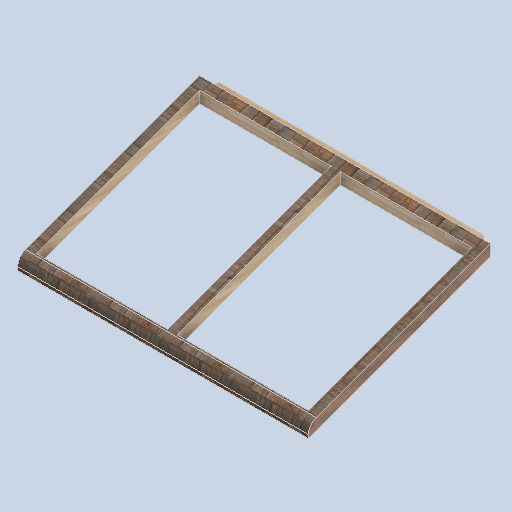
# Autodesk Inventor part: side_curve_frame_02
Saved by Autodesk Inventor 2024.2 (Build 282272000, 272)
## iProperties
Created: 2024-05-24
Part Number: side_curve_frame_02
Material: Wood (Maple)
Document SubType Name: Modeling
Designer: LOSTER_1
Density: 0.67 g/cm^3
Appearance: Natural Maple - Glossy Dark Tint
Author: LOSTER_1
Autodesk Inventor part; units mm, degrees
ref_plane "YZ Plane" through (0, 0, 0) normal (1, 0, 0) x (0, 1, 0)
sketch "Sketch1" plane through (0, 0, 0) normal (0, 0, 1) x (1, 0, 0)
  line L0 (1783.0786, 1495.7799) -> (-1969.0329, 1495.7799)
  line L1 (-1969.0329, 1495.7799) -> (-1969.0329, 1345.7799)
  line L2 (-1969.0329, 1345.7799) -> (1783.0786, 1345.7799)
  line L3 (1783.0786, 1345.7799) -> (1783.0786, 1495.7799)
  point P0 (0, 0)
  point P1 (1784.5139, 676.7735)
  point P2 (1648.0785, 676.7735)
  point P3 (-1769.0329, 888.0934)
  point P4 (-1769.0329, 1496.9217)
  point P5 (-1969.0329, -1503.0783)
  point P6 (-1969.0329, 1496.9217)
  dimension "d0" = 150
  dimension "d7" = 3752.1115
  constraints: 8 end point, 2 parallel, 1 horizontal, 1 perpendicular
  measures "d0" distance of L1.end L0.end
  measures "d7" distance of L0.start L0.end
extrude "Extrusion1" add sketch "Sketch1" along normal blind 50
ref_plane "Work Plane1" through (0, 0, 50) normal (0, 0, 1) x (1, 0, 0)
ref_plane "Work Plane2" through (-1969.0329, 1495.7799, 0) normal (-1, 0, 0) x (0, -1, 0)
sketch "Sketch2" plane through (-1969.0329, 1495.7799, 0) normal (-1, 0, 0) x (0, -1, 0)
  line L0 (0, 50) -> (150, 50)
  line L1 (0, 50) -> (855.0504, 2399.2316)
  line L2 (0, 50) -> (2500, 50) construction
  line L3 (855.0504, 2399.2316) -> (1005.0504, 2399.2316)
  line L4 (1005.0504, 2399.2316) -> (150, 50)
  point P0 (1495.7799, 0)
  dimension "d4" = 2500
  dimension "d5" = 70
  dimension "d6" = 150
  constraints: 10 end point, 3 horizontal, 1 equal length
  measures "d4" distance of L0.start L1.end
  measures "d5" angle of L2 L1
  measures "d6" distance of L1.end L3.end
extrude "Extrusion2" add sketch "Sketch2" against normal blind 3752
sketch "Sketch3" plane through (-1969.0329, 1495.7799, 0) normal (0, 1, 0) x (1, 0, 0)
  line L0 (0, 0) -> (0, -50) projected
  line L1 (200, 0) -> (0, 0)
  line L2 (0, 0) -> (0, -25)
  line L3 (200, -25) -> (200, 0)
  line L4 (3752.1115, 0) -> (3752.1115, -50) projected
  line L5 (3617.1114, 0) -> (3752.1115, 0)
  line L6 (3752.1115, 0) -> (3752.1115, -25)
  line L7 (3617.1114, -25) -> (3617.1114, 0)
  line L8 (3617.1114, -25) -> (3617.1114, -50)
  line L9 (3617.1114, -50) -> (3752.1115, -50)
  line L10 (3752.1115, -25) -> (3752.1115, -50)
  line L11 (0, -50) -> (200, -50)
  line L12 (200, -50) -> (200, -25)
  line L13 (0, -25) -> (0, -50)
  point P0 (1969.0329, 0)
  constraints: 24 end point, 4 perpendicular, 3 horizontal, 3 parallel, 2 midpoint, 1 collinear, 1 vertical
extrude "Extrusion3" cut sketch "Sketch3" against normal through all
sketch "Sketch4" plane through (1782.9671, 1495.7799, 0) normal (1, 0, 0) x (0, 0, -1)
  line L0 (-50, 0) -> (-50, -150) projected
  line L1 (-50, 0) -> (-425.877, -136.8081)
  line L2 (-50, 0) -> (-2399.2316, -855.0504) projected
  line L3 (-425.877, -136.8081) -> (-425.877, -146.8081)
  line L4 (-425.877, -146.8081) -> (-444.6709, -153.6485)
  line L5 (-444.6709, -153.6485) -> (-444.6709, -143.6485)
  line L6 (-444.6709, -143.6485) -> (-820.5479, -280.4565)
  line L7 (-820.5479, -280.4565) -> (-820.5479, -290.4565)
  line L8 (-820.5479, -290.4565) -> (-839.3418, -297.2969)
  line L9 (-839.3418, -297.2969) -> (-839.3418, -287.2969)
  line L10 (-839.3418, -287.2969) -> (-1215.2188, -424.105)
  line L11 (-1215.2188, -424.105) -> (-1215.2188, -434.105)
  line L12 (-1215.2188, -434.105) -> (-1234.0127, -440.9454)
  line L13 (-1234.0127, -440.9454) -> (-1234.0127, -430.9454)
  line L14 (-1234.0127, -430.9454) -> (-1609.8898, -567.7534)
  line L15 (-1609.8898, -567.7534) -> (-1609.2626, -577.5252)
  line L16 (-1609.2626, -577.5252) -> (-1628.0565, -584.3656)
  line L17 (-1628.0565, -584.3656) -> (-1628.6836, -574.5938)
  line L18 (-1628.6836, -574.5938) -> (-2004.5607, -711.4019)
  line L19 (-2004.5607, -711.4019) -> (-2003.9335, -721.1736)
  line L20 (-2003.9335, -721.1736) -> (-2022.7274, -728.014)
  line L21 (-2022.7274, -728.014) -> (-2023.3545, -718.2423)
  line L22 (-2023.3545, -718.2423) -> (-425.877, -136.8081)
  point P0 (0, -1495.7799)
  dimension "d12" = 400
  dimension "d13" = 10
  dimension "d14" = 20
  dimension "d15" = 400
  dimension "d16" = 20
  dimension "d17" = 400
  dimension "d18" = 20
  dimension "d19" = 400
  dimension "d20" = 20
  dimension "d21" = 400
  dimension "d22" = 20
  constraints: 42 end point, 8 parallel, 4 point on line, 3 vertical, 1 collinear, 12 other
  measures "d12" distance of L0.start L1.end
  measures "d13" distance of L1.end L3.end
  measures "d14" distance of L3.end L4.end
  measures "d15" distance of L5.end L6.end
  measures "d16" distance of L7.end L8.end
  measures "d17" distance of L9.end L10.end
  measures "d18" distance of L11.end L12.end
  measures "d19" distance of L13.end L14.end
  measures "d20" distance of L15.end L16.end
  measures "d21" distance of L17.end L18.end
  measures "d22" distance of L19.end L20.end
sketch "Sketch5" plane through (-1769.0329, 1495.7799, 0) normal (0, 1, 0) x (1, 0, 0)
  line L0 (-200, -2399.2316) -> (-200, -50) projected
  line L1 (-200, -2399.2316) -> (3552, -2399.2316) projected
  line L2 (3552, -50) -> (3552, -2399.2316) projected
  line L3 (3552, -50) -> (3417.1114, -50) projected
  line L4 (3417.1114, -50) -> (0, -50) projected
  line L5 (0, -50) -> (-200, -50) projected
  line L6 (-200, -50) -> (-80, -50)
  line L7 (-80, -50) -> (-80, -170)
  line L8 (-80, -170) -> (-200, -170)
  line L9 (-200, -170) -> (-200, -50)
  line L10 (3552, -2399.2316) -> (3432, -2399.2316)
  line L11 (3432, -2399.2316) -> (3432, -2279.2316)
  line L12 (3432, -2279.2316) -> (3552, -2279.2316)
  line L13 (3552, -2279.2316) -> (3552, -2399.2316)
  line L14 (3432, -2279.2316) -> (-80, -2279.2316)
  line L15 (-80, -2279.2316) -> (-80, -170)
  line L16 (-80, -170) -> (3432, -170)
  line L17 (3432, -170) -> (3432, -2279.2316)
  line L18 (1676, -2279.2316) -> (1616, -2279.2316)
  line L19 (1616, -2279.2316) -> (1616, -170)
  line L20 (1616, -170) -> (1676, -170)
  line L21 (1676, -170) -> (1736, -170)
  line L22 (1736, -170) -> (1736, -2279.2316)
  line L23 (1736, -2279.2316) -> (1676, -2279.2316)
  point P0 (1769.0329, 0)
  dimension "d23" = 120
  dimension "d24" = 120
  dimension "d25" = 120
  dimension "d26" = 120
  constraints: 36 end point, 8 parallel, 5 horizontal, 5 perpendicular, 2 midpoint, 2 point on line
  measures "d23" distance of L7.end L8.end
  measures "d24" distance of L6.end L7.end
  measures "d25" distance of L11.end L12.end
  measures "d26" distance of L10.end L11.end
fillet "Fillet1" radius 150 1 edges at (-93.0329, 640.7295, 2399.2316)
extrude "Extrusion5" cut sketch "Sketch5" against normal through all contours L16 L19 L14 L15 | L14 L22 L16 L17
sketch "Sketch6" plane through (-1849.0329, 534.4059, 2279.2316) normal (1, 0, 0) x (0, 0, -1)
  line L0 (0, 150) -> (2109.2316, 917.6975) projected
  line L1 (0, 150) -> (0, 0) projected
  line L2 (2109.2316, 767.6975) -> (0, 0) projected
  line L3 (2109.2316, 917.6975) -> (2109.2316, 767.6975) projected
  point P0 (2279.2316, -534.4059)
body "Solid1"
